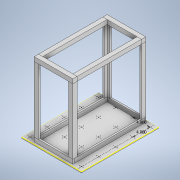
# Autodesk Inventor part: MUDBasePlate
Saved by Autodesk Inventor 2022 (Build 260153000, 153)
## iProperties
Created: 2022-06-07
Part Number: MUDBasePlate
Material: Generic
Document SubType Name: Modeling
Designer: jlwhe
Density: 1 g/cm^3
Appearance: Default
Author: jlwhe
Autodesk Inventor part; units mm, degrees
sketch "BasePlateShapeAndLayout" plane through (0, 0, 0) normal (0, 1, 0) x (-1, 0, 0)
  line L0 (0, 0) -> (355.6, 0)
  line L1 (355.6, 0) -> (355.6, -457.2)
  line L2 (355.6, -457.2) -> (0, -457.2)
  line L3 (0, -457.2) -> (0, 0)
  line L4 (355.6, 0) -> (0, -457.2) construction
  line L5 (355.6, -457.2) -> (0, 0) construction
  line L6 (292.1, -444.5) -> (63.5, -444.5)
  line L7 (63.5, -444.5) -> (63.5, -12.7)
  line L8 (63.5, -12.7) -> (292.1, -12.7)
  line L9 (292.1, -12.7) -> (292.1, -444.5)
  line L10 (292.1, -444.5) -> (63.5, -12.7) construction
  line L11 (63.5, -444.5) -> (292.1, -12.7) construction
  line L12 (282.575, -22.225) -> (73.025, -22.225)
  line L13 (73.025, -22.225) -> (73.025, -434.975)
  line L14 (73.025, -434.975) -> (282.575, -434.975)
  line L15 (282.575, -434.975) -> (282.575, -22.225)
  line L16 (63.5, -173.0375) -> (63.5, -12.7)
  line L17 (292.1, -22.225) -> (292.1, -12.7)
  line L18 (292.1, -12.7) -> (282.575, -12.7)
  line L19 (282.575, -12.7) -> (282.575, -22.225)
  line L20 (282.575, -22.225) -> (292.1, -22.225)
  line L21 (292.1, -22.225) -> (292.1, -12.7)
  line L22 (63.5, -12.7) -> (73.025, -12.7)
  line L23 (73.025, -12.7) -> (73.025, -22.225)
  line L24 (73.025, -22.225) -> (63.5, -22.225)
  line L25 (63.5, -22.225) -> (63.5, -12.7)
  line L26 (73.025, -434.975) -> (63.5, -434.975)
  line L27 (63.5, -434.975) -> (63.5, -444.5)
  line L28 (63.5, -444.5) -> (73.025, -444.5)
  line L29 (73.025, -444.5) -> (73.025, -434.975)
  line L30 (282.575, -434.975) -> (292.1, -434.975)
  line L31 (292.1, -434.975) -> (292.1, -444.5)
  line L32 (292.1, -444.5) -> (282.575, -444.5)
  line L33 (282.575, -444.5) -> (282.575, -434.975)
  line L34 (292.1, -12.7) -> (282.575, -22.225)
  line L35 (63.5, -12.7) -> (73.025, -22.225)
  line L36 (63.5, -444.5) -> (73.025, -434.975)
  line L37 (292.1, -444.5) -> (282.575, -434.975)
  point P0 (177.8, -228.6)
  dimension "d0" = 355.6
  dimension "d1" = 457.2
  dimension "d52" = 228.6
  dimension "d53" = 431.8
  dimension "d54" = 9.525
  constraints: 76 end point, 14 parallel, 10 perpendicular, 6 horizontal, 4 point on line, 3 midpoint, 1 collinear, 3 other
  measures "d0" distance of L1.end L2.end
  measures "d1" distance of L0.end L1.end
  measures "d52" distance of L7.end L8.end
  measures "d53" distance of L6.end L7.end
  measures "d54" distance between parallel lines of L8 L12
extrude "Extrusion1" add sketch "BasePlateShapeAndLayout" against normal blind 6.35 contours L0 L1 L2 L3 | L37 L30 L9 | L6 L33 L37 | L6 L29 L14 L33 | L30 L15 L20 L9 | L14 L13 L12 L15 | L6 L36 L29 | L20 L34 L9 | L26 L7 L24 L13 | L36 L7 L26 | L12 L23 L8 L19 | L19 L8 L34 | L35 L8 L23 | L24 L7 L35
sketch "MountingHoles" plane through (0, 0, 0) normal (0, -1, 0) x (1, 0, 0)
  line L0 (0, -457.2) -> (0, 0) projected
  line L1 (0, 0) -> (-355.6, 0) projected
  line L2 (-25.4, -431.8) -> (-25.4, 0) construction
  line L3 (-25.4, -25.4) -> (-25.4, -457.2) construction
  line L4 (-355.6, -457.2) -> (0, -457.2) construction
  line L5 (-330.2, -431.8) -> (-355.6, -431.8) construction
  line L6 (-355.6, 0) -> (-355.6, -457.2) construction
  line L7 (-25.4, -431.8) -> (0, -431.8) construction
  point P0 (-25.4, -330.2)
  point P1 (-25.4, -228.6)
  point P2 (-25.4, -127)
  point P3 (-127, -431.8)
  point P4 (-127, -330.2)
  point P5 (-127, -228.6)
  point P6 (-127, -127)
  point P7 (-127, -25.4)
  point P8 (-228.6, -431.8)
  point P9 (-228.6, -330.2)
  point P10 (-228.6, -228.6)
  point P11 (-228.6, -127)
  point P12 (-228.6, -25.4)
  point P13 (-330.2, -330.2)
  point P14 (-330.2, -228.6)
  point P15 (-330.2, -127)
  point P16 (-330.2, -25.4)
  dimension "d8" = 101.6
  dimension "d11" = 101.6
  constraints: 8 end point, 5 point on line, 3 perpendicular, 2 collinear, 1 horizontal, 1 vertical, 19 other
  measures "d8" distance of L2.start point (-25.4, -330.2)
  measures "d11" distance of L2.start point (-127, -431.8)
ref_plane "Work Plane6" through (-63.5, 0, -12.7) normal (1, 0, 0) x (0, 0, -1)
ref_plane "Work Plane7" through (-63.5, 0, -22.225) normal (0, 0, 1) x (1, 0, 0)
ref_plane "Work Plane8" through (-63.5, 0, -434.975) normal (0, 0, -1) x (-1, 0, 0)
ref_plane "Work Plane9" through (-292.1, 0, -12.7) normal (-1, 0, 0) x (0, 0, 1)
sketch "Sketch7" plane through (-63.5, 0, -12.7) normal (1, 0, 0) x (0, 0, -1)
  line L0 (0, 0) -> (9.525, 0)
  line L1 (9.525, 0) -> (9.525, 25.4)
  line L2 (9.525, 25.4) -> (0, 25.4)
  line L3 (0, 25.4) -> (0, 0)
  line L4 (431.8, 0) -> (0, 0) projected
  line L5 (215.9, 0) -> (215.9, 19.2581) construction
  line L6 (431.8, 0) -> (422.275, 0)
  line L7 (422.275, 0) -> (422.275, 25.4)
  line L8 (422.275, 25.4) -> (431.8, 25.4)
  line L9 (431.8, 25.4) -> (431.8, 0)
  point P0 (-12.7, 0)
  point P1 (0, 0)
  point P2 (431.8, 0)
  point P3 (422.275, 0)
  dimension "d62" = 9.525
  dimension "d63" = 25.4
  constraints: 18 end point, 6 symmetric about line, 2 parallel, 1 horizontal, 1 midpoint, 1 perpendicular, 1 vertical
  measures "d62" distance of L2.end L1.end
  measures "d63" distance of L1.end L0.end
sketch "Sketch8" plane through (-63.5, 0, -22.225) normal (0, 0, 1) x (1, 0, 0)
  line L0 (0, 0) -> (-9.525, 0)
  line L1 (-9.525, 0) -> (-9.525, 25.4)
  line L2 (-9.525, 25.4) -> (0, 25.4)
  line L3 (0, 25.4) -> (0, 0)
  line L4 (-114.3, 0) -> (-114.3, 16.4265) construction
  line L5 (-228.6, 0) -> (-219.075, 0)
  line L6 (-219.075, 0) -> (-219.075, 25.4)
  line L7 (-219.075, 25.4) -> (-228.6, 25.4)
  line L8 (-228.6, 25.4) -> (-228.6, 0)
  point P0 (63.5, 0)
  point P1 (0, 0)
  point P2 (-228.6, 0)
  dimension "d64" = 9.525
  dimension "d65" = 25.4
  constraints: 18 end point, 6 symmetric about line, 2 parallel, 1 horizontal, 1 perpendicular, 1 vertical
  measures "d64" distance of L1.end L2.end
  measures "d65" distance of L0.end L1.end
extrude "Extrusion9" add sketch "Sketch7" against normal up to surface (228.6 mm away) separate body contours L3 L2 L1 L0
extrude "Extrusion10" add sketch "Sketch7" against normal up to surface (228.6 mm away) separate body contours L7 L8 L9 L4
extrude "Extrusion11" add sketch "Sketch8" against normal up to surface (412.75 mm away) separate body contours L0 L1 L2 L3
extrude "Extrusion12" add sketch "Sketch8" against normal up to surface (412.75 mm away) separate body contours L8 L7 L6 L5
sketch "Sketch9" plane through (-63.5, 25.4, -12.7) normal (0, 1, 0) x (1, 0, 0)
  line L0 (0, 9.525) -> (0, 0) projected
  line L1 (0, 0) -> (-25.4, 0)
  line L2 (-25.4, 0) -> (-25.4, 25.4)
  line L3 (-25.4, 25.4) -> (0, 25.4)
  line L4 (0, 25.4) -> (0, 0)
  line L5 (-25.4, 9.525) -> (-9.525, 9.525)
  line L6 (-114.3, 215.9) -> (-110.8317, 215.9) construction
  line L7 (-114.3, 215.9) -> (-114.3, 210.2054) construction
  line L8 (-9.525, 9.525) -> (-9.525, 25.4)
  line L9 (-228.6, 9.525) -> (-228.6, 0)
  line L10 (-228.6, 0) -> (-203.2, 0)
  line L11 (-203.2, 0) -> (-203.2, 25.4)
  line L12 (-203.2, 25.4) -> (-228.6, 25.4)
  line L13 (-228.6, 25.4) -> (-228.6, 0)
  line L14 (-203.2, 9.525) -> (-219.075, 9.525)
  line L15 (-219.075, 9.525) -> (-219.075, 25.4)
  line L16 (0, 422.275) -> (0, 431.8)
  line L17 (0, 431.8) -> (-25.4, 431.8)
  line L18 (-25.4, 431.8) -> (-25.4, 406.4)
  line L19 (-25.4, 406.4) -> (0, 406.4)
  line L20 (0, 406.4) -> (0, 431.8)
  line L21 (-25.4, 422.275) -> (-9.525, 422.275)
  line L22 (-9.525, 422.275) -> (-9.525, 406.4)
  line L23 (-228.6, 422.275) -> (-228.6, 431.8)
  line L24 (-228.6, 431.8) -> (-203.2, 431.8)
  line L25 (-203.2, 431.8) -> (-203.2, 406.4)
  line L26 (-203.2, 406.4) -> (-228.6, 406.4)
  line L27 (-228.6, 406.4) -> (-228.6, 431.8)
  line L28 (-203.2, 422.275) -> (-219.075, 422.275)
  line L29 (-219.075, 422.275) -> (-219.075, 406.4)
  point P0 (63.5, -12.7)
  point P1 (-9.525, 9.525)
  point P2 (0, 9.525)
  point P3 (-219.075, 9.525)
  dimension "d74" = 25.4
  dimension "d75" = 25.4
  dimension "d76" = 9.525
  dimension "d86" = 9.525
  constraints: 58 end point, 27 symmetric about line, 8 point on line, 3 coincident, 3 horizontal, 3 perpendicular, 2 parallel, 1 vertical, 9 other
  measures "d74" distance of L2.end L3.end
  measures "d75" distance of L1.end L2.end
  measures "d76" distance between parallel lines of L5 L1
  measures "d86" distance between parallel lines of L8 L4
extrude "Extrusion13" add sketch "Sketch9" along normal blind 387.35 separate body contours L0 L1 L2 L5 L8 L3 L4
extrude "Extrusion14" add sketch "Sketch9" along normal blind 387.35 separate body contours L13 L12 L15 L14 L11 L10 L9
extrude "Extrusion15" add sketch "Sketch9" along normal blind 387.35 separate body contours L23 L24 L25 L28 L29 L26 L27
extrude "Extrusion16" add sketch "Sketch9" along normal blind 387.35 separate body contours L20 L19 L22 L21 L18 L17 L16
sketch "Sketch10" plane through (-63.5, 25.4, -12.7) normal (1, 0, 0) x (0, 0, -1)
  line L0 (0, 387.35) -> (25.4, 387.35) projected
  line L1 (0, 387.35) -> (25.4, 387.35)
  line L2 (25.4, 387.35) -> (25.4, 412.75)
  line L3 (25.4, 412.75) -> (0, 412.75)
  line L4 (0, 412.75) -> (0, 387.35)
  line L5 (215.9, -25.4) -> (215.9, 31.6013) construction
  line L6 (431.8, 387.35) -> (406.4, 387.35)
  line L7 (431.8, 387.35) -> (406.4, 387.35)
  line L8 (406.4, 387.35) -> (406.4, 412.75)
  line L9 (406.4, 412.75) -> (431.8, 412.75)
  line L10 (431.8, 412.75) -> (431.8, 387.35)
  point P0 (-12.7, -25.4)
  dimension "d87" = 25.4
  dimension "d88" = 25.4
  constraints: 20 end point, 5 symmetric about line, 2 parallel, 1 horizontal, 1 perpendicular, 1 vertical
  measures "d87" distance of L3.end L2.end
  measures "d88" distance of L2.end L1.end
sketch "Sketch11" plane through (-63.5, 25.4, -38.1) normal (0, 0, -1) x (-1, 0, 0)
  line L0 (0, 387.35) -> (25.4, 387.35)
  line L1 (25.4, 387.35) -> (25.4, 412.75)
  line L2 (25.4, 412.75) -> (0, 412.75)
  line L3 (0, 412.75) -> (0, 387.35)
  line L4 (114.3, -25.4) -> (114.3, -19.7607) construction
  line L5 (228.6, 387.35) -> (203.2, 387.35)
  line L6 (203.2, 387.35) -> (203.2, 412.75)
  line L7 (203.2, 412.75) -> (228.6, 412.75)
  line L8 (228.6, 412.75) -> (228.6, 387.35)
  point P0 (-63.5, -25.4)
  dimension "d89" = 25.4
  dimension "d90" = 25.4
  constraints: 18 end point, 4 symmetric about line, 2 parallel, 1 horizontal, 1 perpendicular, 1 vertical
  measures "d89" distance of L2.end L1.end
  measures "d90" distance of L1.end L0.end
extrude "Extrusion17" add sketch "Sketch10" against normal up to surface (228.6 mm away) separate body contours L4 L3 L2 L0
extrude "Extrusion18" add sketch "Sketch10" against normal up to surface (228.6 mm away) separate body contours L6 L8 L9 L10
extrude "Extrusion19" add sketch "Sketch11" along normal up to surface (381 mm away) separate body contours L3 L2 L1 L0
extrude "Extrusion20" add sketch "Sketch11" along normal up to surface (381 mm away) separate body contours L5 L6 L7 L8
equation "\"d62\" = d76"
equation "\"d64\" = d54"
equation "\"d65\" = d63"
equation "\"d74\" = d63"
equation "\"d75\" = d63"
equation "\"d86\" = d76"
equation "\"d87\" = d63"
equation "\"d88\" = d63"
equation "\"d89\" = d63"
equation "\"d90\" = d63"
body "Solid7"
body "Solid8"
body "Solid9"
body "Solid10"
body "Solid11"
body "Solid12"
body "Solid13"
body "Solid14"
body "Solid15"
body "Solid16"
body "Solid17"
body "Solid18"
